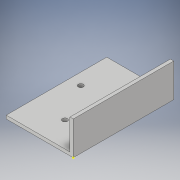
# Autodesk Inventor part: モーター固定
Saved by Autodesk Inventor 2019 (Build 230136000, 136)
## iProperties
Created: 2018-09-25
Part Number: モーター固定
Material: 一般
Document SubType Name: Modeling
Designer: kouki
Density: 1 g/cm^3
Appearance: 既定
Author: kouki
Autodesk Inventor part; units mm, degrees
ref_plane "YZ Plane" through (0, 0, 0) normal (1, 0, 0) x (0, 1, 0)
ref_plane "XZ Plane" through (0, 0, 0) normal (0, 1, 0) x (-1, 0, 0)
ref_plane "XY Plane" through (0, 0, 0) normal (0, 0, 1) x (1, 0, 0)
sketch "スケッチ1" plane through (0, 0, 0) normal (0, 1, 0) x (-1, 0, 0)
  line L0 (0, 0) -> (40, 0)
  line L1 (40, 0) -> (40, -60)
  line L2 (40, -60) -> (0, -60)
  line L3 (0, -60) -> (0, 0)
  dimension "d0" = 40
  dimension "d1" = 60
  constraints: 8 end point, 2 parallel, 1 horizontal, 1 perpendicular
  measures "d0" distance of L1.end L2.end
  measures "d1" distance of L1.end L0.end
extrude "押し出し1" add sketch "スケッチ1" along normal blind 2
sketch "スケッチ2" plane through (0, 0, 0) normal (1, 0, 0) x (0, 0, -1)
  line L0 (0, 2) -> (60, 2)
  line L1 (60, 2) -> (60, 30)
  line L2 (60, 30) -> (0, 30)
  line L3 (0, 30) -> (0, 2)
  point P0 (0, 0)
  dimension "d4" = 60
  dimension "d5" = 28
  constraints: 8 end point, 2 parallel, 1 horizontal, 1 perpendicular
  measures "d4" distance of L2.end L1.end
  measures "d5" distance of L1.end L0.end
extrude "押し出し2" add sketch "スケッチ2" against normal blind 2
sketch "スケッチ5" plane through (0, 0, 0) normal (1, 0, 0) x (0, 0, -1)
  point P0 (0, 0)
sketch "スケッチ9" plane through (0, 0, 0) normal (0, -1, 0) x (1, 0, 0)
  point P0 (0, 0)
sketch "スケッチ11" plane through (0, 30, 0) normal (0, 1, 0) x (1, 0, 0)
  line L0 (0, 0) -> (-2, 0)
  line L1 (-2, 0) -> (-2, 60)
  line L2 (-2, 60) -> (0, 60)
  line L3 (0, 60) -> (0, 0)
  constraints: 8 end point, 2 parallel, 1 horizontal, 1 perpendicular
extrude "押し出し6" cut sketch "スケッチ11" against normal blind 10
sketch "スケッチ12" plane through (0, 0, 0) normal (0, -1, 0) x (1, 0, 0)
  line L0 (0, -60) -> (0, 0) projected
  line L1 (0, -30) -> (-14, -30)
  dimension "d67" = 14
  constraints: 2 end point, 1 coincident, 1 horizontal, 1 midpoint
  measures "d67" distance of L1.start L1.end
hole "穴4" at (-14, 0, -30) direction (0, 1, 0) diameter 12 end through all
sketch "スケッチ13" plane through (0, 0, 0) normal (0, -1, 0) x (1, 0, 0)
  line L0 (0, -60) -> (0, 0) projected
  line L1 (0, -30) -> (-20, -30)
  circle A0 centre (-20, -30) radius 15
  line L2 (-20, -30) -> (-20, -15)
  line L3 (-20, -30) -> (5.9808, -45)
  line L4 (-20, -30) -> (-149.9038, -105)
  point P0 (-7.0096, -37.5)
  point P1 (-32.9904, -37.5)
  dimension "d76" = 30
  dimension "d75" = 20
  dimension "d77" = 15
  dimension "d78" = 30
  dimension "d79" = 150
  dimension "d80" = 120
  dimension "d81" = 120
  constraints: 8 end point, 3 coincident, 2 midpoint, 1 horizontal, 1 point on line, 1 vertical, 3 other
  measures "d75" distance of L1.start L1.end
  measures "d77" distance of L2.start L2.end
  measures "d78" distance of L2.start L3.end
  measures "d79" distance of L2.start L4.end
  measures "d80" angle of L4 L2
  measures "d81" angle of L3 L2
hole "穴5" at (-7.0096, 0, -37.5) at (-32.9904, 0, -37.5) at (-20, 0, -15) direction (0, 1, 0) diameter 3 end through all
